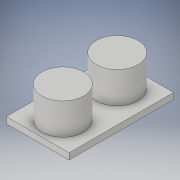
# Autodesk Inventor part: Ultraschallsensor
Saved by Autodesk Inventor 2019.5 (Build 235369000, 369)
## iProperties
Created: 2021-09-30
Part Number: Ultraschallsensor
Material: Generisch
Document SubType Name: Modeling
Designer: mritt
Density: 1 g/cm^3
Appearance: Vorgabe
Author: mritt
Autodesk Inventor part; units mm, degrees
ref_plane "YZ Plane" through (0, 0, 0) normal (1, 0, 0) x (0, 1, 0)
ref_plane "XZ Plane" through (0, 0, 0) normal (0, 1, 0) x (-1, 0, 0)
ref_plane "XY Plane" through (0, 0, 0) normal (0, 0, 1) x (1, 0, 0)
sketch "Skizze1" plane through (0, 0, 0) normal (0, 1, 0) x (-1, 0, 0)
  line L0 (45.2756, -27.3622) -> (15.2756, -27.3622)
  line L1 (15.2756, -27.3622) -> (15.2756, -77.3622)
  line L2 (15.2756, -77.3622) -> (45.2756, -77.3622)
  line L3 (45.2756, -77.3622) -> (45.2756, -27.3622)
  point P0 (0, 0)
  dimension "d0" = 50
  dimension "d1" = 30
  constraints: 8 end point, 2 parallel, 1 horizontal, 1 perpendicular
  measures "d0" distance of L2.end L0.start
  measures "d1" distance of L1.end L2.end
extrude "Extrusion1" add sketch "Skizze1" along normal blind 3
sketch "Skizze2" plane through (0, 3, 0) normal (0, 1, 0) x (1, 0, 0)
  circle A0 centre (-30.2756, 39.3622) radius 10
  circle A1 centre (-30.2756, 65.3622) radius 10
  line L0 (-45.2756, 77.3622) -> (-45.2756, 27.3622) projected
  line L1 (-45.2756, 27.3622) -> (-15.2756, 27.3622) projected
  line L2 (-15.2756, 77.3622) -> (-45.2756, 77.3622) projected
  point P0 (0, 0)
  dimension "d4" = 20
  dimension "d5" = 20
  dimension "d6" = 15
  dimension "d7" = 15
  dimension "d10" = 12
  dimension "d11" = 12
  constraints: 2 centre point
  measures "d4" diameter of A0
  measures "d5" diameter of A1
  measures "d6" distance from line of A0.centre L0
  measures "d7" distance from line of A1.centre L0
  measures "d10" distance from line of A0.centre L1
  measures "d11" distance from line of A1.centre L2
extrude "Extrusion2" add sketch "Skizze2" along normal blind 15
